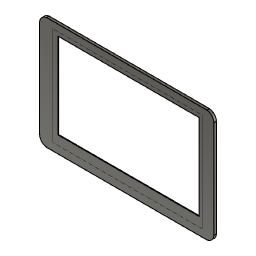
Display_Bezel v3 (Autodesk Fusion 360 design; units mm, degrees)
Autodesk Fusion 360 part; units mm, degrees
note: some values were not read from the file. Set by a fixed rule: which face or edge a step refers to.
sketch "Sketch8" plane through (0, -3.5, 0) normal (0, -1, 0) x (1, 0, 0)
  line L0 (3.9555, -0.4058) -> (3.9555, 77.5942)
  line L1 (3.9555, 77.5942) -> (122.4555, 77.5942)
  line L2 (122.4555, 77.5942) -> (122.4555, -0.4058)
  line L3 (122.4555, -0.4058) -> (3.9555, -0.4058)
  circle A0 centre (126, 0) radius 2
  circle A1 centre (126, 77) radius 2
  circle A2 centre (0, 77) radius 2
  circle A3 centre (0, 0) radius 2
  line L4 (-6, -6) -> (132, -6)
  line L5 (132, 83) -> (-6, 83)
  line L6 (8.57, 74.76) -> (120.31, 74.76)
  line L7 (120.31, 74.76) -> (120.31, 7.08)
  line L8 (120.31, 7.08) -> (8.57, 7.08)
  line L9 (8.57, 7.08) -> (8.57, 74.76)
  line L10 (0, 77) -> (-5.9998, 77.0479) construction
  line L11 (0, 0) -> (-6, 0) construction
  arc A4 (0.2349, 83.0347) -> (-5.9998, 77.0479) centre (0.2349, 76.7949) ccw
  line L12 (63, 83) -> (63, -6) construction
  line L13 (-16, 38.5) -> (142, 38.5) construction
  arc A5 (-5.9998, -0.0479) -> (0.2349, -6.0347) centre (0.2349, 0.2051) ccw
  line L14 (-5.9998, 77.0479) -> (-5.9998, -0.0479)
  line L15 (131.9998, 77.0479) -> (131.9998, -0.0479)
  arc A6 (131.9998, 77.0479) -> (125.7651, 83.0347) centre (125.7651, 76.7949) ccw
  arc A7 (125.7651, -6.0347) -> (131.9998, -0.0479) centre (125.7651, 0.2051) ccw
  line L16 (0.2349, 83.0347) -> (125.7651, 83.0347)
  line L17 (0.2349, -6.0347) -> (125.7651, -6.0347)
  line L18 (3.9555, 77.5942) -> (122.4555, 77.5942)
  line L19 (122.4555, 77.5942) -> (122.4555, -0.4058)
  line L20 (122.4555, -0.4058) -> (3.9555, -0.4058)
  line L21 (3.9555, -0.4058) -> (3.9555, 77.5942)
  line L22 (-6, 83) -> (-6, -6)
  line L23 (132, -6) -> (132, 83)
  dimension "d54" = 6
  dimension "d55" = 6
  constraint horizontal L6
  constraint vertical L7
  constraint horizontal L8
  constraint vertical L9
  constraint coincident A2.centre L10.start
  constraint coincident A3.centre L11.start
  constraint midpoint L5 L12.start
  constraint symmetric L10.end L13 A5.start
  constraint symmetric A4.start L13 A5.end
  constraint symmetric A4 L13 A5
  constraint symmetric L10.end L12 L15.start
  constraint symmetric A4.start L12 A6.end
  constraint symmetric A4 L12 A6
  constraint symmetric L12 A5.end A7.start
  constraint symmetric L12 A5.start L15.end
  constraint symmetric L12 A5 A7
  constraint tangent A6 L16
  constraint tangent A7 L17
  constraint horizontal L18
  constraint vertical L19
  constraint horizontal L20
  constraint vertical L21
  constraint coincident L2.end L3.start
  constraint coincident L0.end L1.start
  measures "d54" distance of A2.centre L10.end
  measures "d55" distance of A3.centre L11.end
extrude "Extrude9" add sketch "Sketch8" along normal blind 1 contours L0 L1 L2 L3 L18 L19 L20 L21 | A0 | A1 | A2 | A3 | L4 L5 A4 A5 L14 L15 A6 A7 L22 L23
extrude "Extrude10" add sketch "Sketch8" against normal blind 1 contours L4 L5 A4 A5 L14 L15 A6 A7 L22 L23
sketch "Sketch10" plane through (0, -2.5, 0) normal (0, 1, 0) x (-1, 0, 0)
  circle A0 centre (-126, 0) radius 2
  circle A1 centre (0, 0) radius 2
  line L0 (-3.9555, -0.4058) -> (-122.4555, -0.4058)
  line L1 (-122.4555, -0.4058) -> (-122.4555, 77.5942)
  line L2 (-122.4555, 77.5942) -> (-3.9555, 77.5942)
  line L3 (-3.9555, 77.5942) -> (-3.9555, -0.4058)
  circle A2 centre (-126, 77) radius 2
  circle A3 centre (0, 77) radius 2
  arc A4 (-126.4223, 83) -> (-131.9998, 77.0479) centre (-125.7651, 76.7949) ccw
  line L4 (-131.9998, 77.0479) -> (-131.9998, -0.0479)
  arc A5 (-131.9998, -0.0479) -> (-126.4223, -6) centre (-125.7651, 0.2051) ccw
  line L5 (-126.4223, -6) -> (0.4223, -6)
  arc A6 (0.4223, -6) -> (5.9998, -0.0479) centre (-0.2349, 0.2051) ccw
  line L6 (5.9998, -0.0479) -> (5.9998, 77.0479)
  arc A7 (5.9998, 77.0479) -> (0.4223, 83) centre (-0.2349, 76.7949) ccw
  line L7 (0.4223, 83) -> (-126.4223, 83)
  circle A8 centre (0, 0) radius 3.5
  circle A9 centre (-126, 0) radius 3.5
  circle A10 centre (-126, 77) radius 3.5
  circle A11 centre (0, 77) radius 3.5
  dimension "d63" = 7
  dimension "d64" = 7
  dimension "d65" = 7
  dimension "d66" = 7
  constraint concentric A1 A8
  constraint concentric A0 A9
  constraint concentric A2 A10
  constraint concentric A3 A11
  measures "d63" diameter of A8
  measures "d64" diameter of A9
  measures "d65" diameter of A10
  measures "d66" diameter of A11
extrude "Extrude12" cut sketch "Sketch10" against normal blind 0.5 contours A8 | A9 | A10 | A11
move_face "OffsetFaces1" offset -0.5 20 faces at (0.5251, -3.5, 77.9392) (44.9937, -3.5, 2.0894) (125.6568, -3.5, 76.3794) (-0.3955, -3.5, 0.2516) (127.3259, -3.5, -0.0994) (0.5251, -3.5, 77.9392) (44.9937, -3.5, 2.0894) (125.6568, -3.5, 76.3794) (-0.3955, -3.5, 0.2516) (127.3259, -3.5, -0.0994) (0.5251, -3.5, 77.9392) (44.9937, -3.5, 2.0894) (125.6568, -3.5, 76.3794) (-0.3955, -3.5, 0.2516) (127.3259, -3.5, -0.0994) (0.5251, -3.5, 77.9392) (44.9937, -3.5, 2.0894) (125.6568, -3.5, 76.3794) (-0.3955, -3.5, 0.2516) (127.3259, -3.5, -0.0994)
sketch "Sketch11" plane through (0, -4, 0) normal (0, 1, 0) x (-1, 0, 0)
  circle A0 centre (-126, 77) radius 2
  circle A1 centre (-126, 77) radius 2
  circle A2 centre (0, 77) radius 2
  circle A3 centre (0, 77) radius 2
  circle A4 centre (0, 0) radius 2
  circle A5 centre (-126, 0) radius 2
  circle A6 centre (-126, 0) radius 2
  point P0 (-124, 77)
  point P1 (2, 77)
  point P2 (2, 0)
  point P3 (-124, 0)
  constraint concentric A0 A1
  constraint coincident A1 P0
  constraint concentric A2 A3
  constraint coincident A2 P1
  constraint coincident A4.centre origin
  constraint coincident A4 P2
  constraint concentric A5 A6
  constraint coincident A5 P3
extrude "Extrude13" add sketch "Sketch11" along normal blind 1
